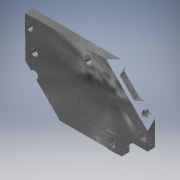
# Autodesk Inventor part: VERTICAL PLATE
Saved by Autodesk Inventor 2016 Beta3 (Build 200134000, 134) ContinuousBuild 0
## iProperties
Created: 2004-06-15
Part Number: VERTICAL PLATE
Document SubType Name: Modeling
Manufacturer: Standard
Standards Organization: Custom
Material: Steel, Mild
Density: 7.86 g/cm^3
Mass: 3865.22 g
Surface Area: 833.818 cm^2
Volume: 491.758 cm^3
Appearance: Steel Galvanized
Author: Autodesk, Inc.
Autodesk Inventor part; units mm, degrees
ref_plane "YZ Plane" through (0, 0, 0) normal (1, 0, 0) x (0, 1, 0)
ref_plane "XZ Plane" through (0, 0, 0) normal (0, 1, 0) x (-1, 0, 0)
ref_plane "XY Plane" through (0, 0, 0) normal (0, 0, 1) x (1, 0, 0)
sketch "Sketch1" plane through (0, 0, 0) normal (0, 0, 1) x (1, 0, 0)
  line L0 (-123.35, 77) -> (123.35, 77)
  line L1 (123.35, 77) -> (123.35, -77)
  line L2 (123.35, -77) -> (-123.35, -77)
  line L3 (-123.35, -77) -> (-123.35, 77)
  point P0 (0, 0)
  point P1 (-123.35, 0)
  point P2 (0, 77)
  dimension "d0" = 246.7
  dimension "d1" = 154
  constraints: 8 end point, 2 midpoint, 2 parallel, 1 horizontal, 1 horizontal alignment, 1 perpendicular, 1 vertical alignment
  measures "d0" distance of L0.start L0.end
  measures "d1" distance of L0.end L1.end
extrude "Extrusion1" add sketch "Sketch1" along normal blind 15
sketch "Sketch2" plane through (0, 0, 15) normal (0, 0, 1) x (1, 0, 0)
  line L0 (-123.35, 77) -> (123.35, 77) projected
  line L1 (123.35, 77) -> (123.35, -77) projected
  line L2 (62.65, 77) -> (62.65, 28.2)
  line L3 (62.65, 28.2) -> (123.35, 28.2)
  line L4 (123.35, -77) -> (-123.35, -77) projected
  line L5 (62.65, 58.2) -> (92.65, 28.2)
  dimension "d4" = 60.7
  dimension "d5" = 105.2
  dimension "d6" = 45
  dimension "d7" = 30.7
  constraints: 6 end point, 4 point on line, 2 perpendicular
  measures "d4" distance between parallel lines of L1 L2
  measures "d5" distance between parallel lines of L3 L4
  measures "d6" angle of L5 L3
  measures "d7" distance from line of L1 L5.end
extrude "Extrusion2" cut sketch "Sketch2" against normal through all contours L0 L1 L3 L5 L2
sketch "Sketch3" plane through (0, 0, 15) normal (0, 0, 1) x (1, 0, 0)
  line L0 (123.35, 28.2) -> (123.35, -77) projected
  line L1 (123.35, -42.45) -> (92.65, -42.45)
  line L2 (92.65, -42.45) -> (71.05, -64.05)
  line L3 (71.05, -64.05) -> (71.05, -77)
  line L4 (123.35, -77) -> (-123.35, -77) projected
  point P0 (92.65, 28.2)
  point P1 (62.65, 58.2)
  dimension "d10" = 34.55
  dimension "d11" = 45
  dimension "d41" = 52.3
  constraints: 6 end point, 2 perpendicular, 2 point on line, 1 vertical alignment
  measures "d10" distance between parallel lines of L4 L1
  measures "d11" angle of L1 L2
  measures "d41" distance between parallel lines of L0 L3
extrude "Extrusion3" cut sketch "Sketch3" against normal through all
fillet "Fillet1" radius 6.35 4 edges at (62.65, 58.2, 7.5) (92.65, 28.2, 7.5) (92.65, -42.45, 7.5) (71.05, -64.05, 7.5)
sketch "Sketch4" plane through (0, 0, 15) normal (0, 0, 1) x (1, 0, 0)
  line L0 (-123.35, 77) -> (-103.35, 77)
  line L1 (-103.35, 77) -> (-103.35, 40)
  line L2 (-103.35, 40) -> (-123.35, 40)
  line L3 (-123.35, 40) -> (-123.35, 77)
  dimension "d15" = 37
  dimension "d16" = 20
  constraints: 8 end point, 2 parallel, 1 horizontal, 1 perpendicular
  measures "d15" distance from line of L0.start L2
  measures "d16" distance of L0.start L0.end
extrude "Extrusion4" add sketch "Sketch4" along normal blind 1
sketch "Sketch5" plane through (0, 0, 16) normal (0, 0, 1) x (1, 0, 0)
  line L0 (-119.35, 55.5) -> (-119.35, 61.5)
  arc A0 (-107.35, 61.5) -> (-119.35, 61.5) centre (-113.35, 61.5) ccw
  line L1 (-107.35, 61.5) -> (-107.35, 55.5)
  arc A1 (-119.35, 55.5) -> (-107.35, 55.5) centre (-113.35, 55.5) ccw
  line L2 (-119.35, 58.5) -> (-107.35, 58.5) construction
  line L3 (-103.35, 77) -> (-103.35, 40) construction
  line L4 (-103.35, 40) -> (-123.35, 40) construction
  point P0 (-103.35, 58.5)
  point P1 (-113.35, 40)
  point P2 (-113.35, 58.5)
  dimension "d23" = 12
  dimension "d24" = 18
  constraints: 6 end point, 5 midpoint, 4 point on circle, 4 tangent, 2 centre point, 1 horizontal alignment, 1 parallel, 1 vertical, 1 vertical alignment
  measures "d23" distance between parallel lines of L1 L0
extrude "Extrusion5" cut sketch "Sketch5" against normal through all
pattern_linear "Rectangular Pattern1" count 2 spacing 118 along (1, 0, 0) of "Extrusion4", "Extrusion5"
sketch "Sketch6" plane through (0, 0, 15) normal (0, 0, 1) x (1, 0, 0)
  line L0 (-123.35, -77) -> (-103.35, -77)
  line L1 (-103.35, -77) -> (-103.35, -44.4)
  line L2 (-103.35, -44.4) -> (-123.35, -44.4)
  line L3 (-123.35, -44.4) -> (-123.35, -77)
  point P0 (-103.35, 40)
  dimension "d30" = 32.6
  constraints: 8 end point, 2 parallel, 1 horizontal, 1 perpendicular, 1 vertical alignment
  measures "d30" distance of L2.end L0.start
extrude "Extrusion6" add sketch "Sketch6" along normal blind 1
sketch "Sketch7" plane through (0, -119.2, 16) normal (0, 0, 1) x (1, 0, 0)
  line L0 (-119.35, 55.5) -> (-119.35, 61.5)
  arc A0 (-107.35, 61.5) -> (-119.35, 61.5) centre (-113.35, 61.5) ccw
  line L1 (-107.35, 61.5) -> (-107.35, 55.5)
  arc A1 (-119.35, 55.5) -> (-107.35, 55.5) centre (-113.35, 55.5) ccw
  line L2 (-119.35, 58.5) -> (-107.35, 58.5) construction
  line L3 (-103.35, 77) -> (-103.35, 40) construction
  line L4 (-103.35, 40) -> (-123.35, 40) construction
  point P0 (-103.35, 58.5)
  point P1 (-113.35, 40)
  point P2 (-113.35, 58.5)
  dimension "d34" = 12
  dimension "d33" = 18
  constraints: 10 end point, 5 midpoint, 4 point on circle, 4 tangent, 2 centre point, 1 horizontal alignment, 1 parallel, 1 vertical, 1 vertical alignment
  measures "d34" distance between parallel lines of L1 L0
extrude "Extrusion7" cut sketch "Sketch7" against normal through all
pattern_linear "Rectangular Pattern2" count 2 spacing 166 along (1, 0, 0) of "Extrusion7", "Extrusion6"
hole "Hole1" at (-105.35, -22.45, 15) direction (0, 0, -1) diameter 8.8 end through all counterbore diameter 15 counterbore depth 9
pattern_linear "Rectangular Pattern3" count 2 spacing 39.13 along (0, 1, 0) count 2 spacing 219.2 along (1, 0, 0) of "Hole1"
body "Solid1"
